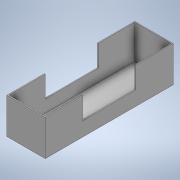
# Autodesk Inventor part: Suport motor superior
Saved by Autodesk Inventor 2021 (Build 250183000, 183)
## iProperties
Created: 2021-03-02
Part Number: Suport motor superior
Material: Plástico ABS
Document SubType Name: Modeling
Designer: Marc
Density: 1.06 g/cm^3
Appearance: Suave - Blanco
Author: Marc
Autodesk Inventor part; units mm, degrees
ref_plane "YZ Plane" through (0, 0, 0) normal (1, 0, 0) x (0, 1, 0)
ref_plane "XZ Plane" through (0, 0, 0) normal (0, 1, 0) x (-1, 0, 0)
ref_plane "XY Plane" through (0, 0, 0) normal (0, 0, 1) x (1, 0, 0)
sketch "Boceto1" plane through (0, 0, 0) normal (0, 1, 0) x (-1, 0, 0)
  line L0 (26.75, 89.25) -> (-26.75, 89.25)
  line L1 (-26.75, 89.25) -> (-26.75, -89.25)
  line L2 (-26.75, -89.25) -> (26.75, -89.25)
  line L3 (26.75, -89.25) -> (26.75, 89.25)
  line L4 (26.75, 89.25) -> (-26.75, -89.25) construction
  line L5 (-26.75, 89.25) -> (26.75, -89.25) construction
  point P0 (0, 0)
  dimension "d0" = 53.5
  dimension "d1" = 178.5
  constraints: 12 end point, 2 midpoint, 2 parallel, 1 horizontal, 1 perpendicular
  measures "d0" distance of L2.end L1.end
  measures "d1" distance of L1.end L0.end
extrude "Extrusión1" add sketch "Boceto1" along normal blind 50
sketch "Boceto2" plane through (0, 50, 0) normal (0, 1, 0) x (1, 0, 0)
  line L0 (-25.5, -88) -> (25.5, -88)
  line L1 (25.5, -88) -> (25.5, 88)
  line L2 (25.5, 88) -> (-25.5, 88)
  line L3 (-25.5, 88) -> (-25.5, -88)
  line L4 (-25.5, -88) -> (25.5, 88) construction
  line L5 (25.5, -88) -> (-25.5, 88) construction
  point P0 (0, 0)
  dimension "d4" = 51
  dimension "d5" = 176
  constraints: 12 end point, 2 midpoint, 2 parallel, 1 horizontal, 1 perpendicular
  measures "d4" distance of L2.end L1.end
  measures "d5" distance of L1.end L0.end
extrude "Extrusión2" cut sketch "Boceto2" against normal blind 47.5
sketch "Boceto3" plane through (26.75, 0, 89.25) normal (1, 0, 0) x (0, 0, -1)
  line L0 (52.25, 50) -> (52.25, 20)
  line L1 (0, 0) -> (178.5, 0) projected
  line L2 (126.25, 50) -> (126.25, 20)
  line L3 (126.25, 20) -> (52.25, 20)
  line L4 (52.25, 50) -> (126.25, 50)
  point P0 (89.25, 0)
  point P1 (177.25, 50)
  point P2 (1.25, 50)
  dimension "d9" = 30
  constraints: 8 end point, 2 perpendicular, 1 horizontal
  measures "d9" distance of L0.start L0.end
extrude "Extrusión3" cut sketch "Boceto3" against normal through all
